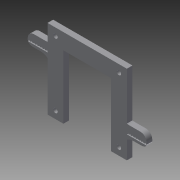
# Autodesk Inventor part: x carriage belt tensioner
Saved by Autodesk Inventor 2014 SP1 (Build 180222100, 222)
## iProperties
Created: 2014-10-23
Part Number: x carriage belt tensioner
Material: Generic
Document SubType Name: Modeling
Designer: Mon
Density: 1 g/cm^3
Appearance: Default
Author: Mon
Autodesk Inventor part; units mm, degrees
ref_plane "YZ Plane" through (0, 0, 0) normal (1, 0, 0) x (0, 1, 0)
ref_plane "XZ Plane" through (0, 0, 0) normal (0, 1, 0) x (-1, 0, 0)
ref_plane "XY Plane" through (0, 0, 0) normal (0, 0, 1) x (1, 0, 0)
sketch "Sketch1" plane through (0, 0, 0) normal (0, 1, 0) x (-1, 0, 0)
  line L0 (15.8278, -0.0229) -> (15.8278, 14.2578)
  arc A0 (15.8278, 14.2578) -> (10.4826, 16.0171) centre (10.4826, 7.0171) ccw
  line L1 (10.4826, 16.0171) -> (4.0229, 16.0171)
  arc A1 (0.0229, 18.0171) -> (4.0229, 16.0171) centre (4.0229, 21.0171) ccw
  line L2 (0.0229, 18.0171) -> (15.8278, 18.0171)
  line L3 (15.8278, 18.0171) -> (15.8278, 18.7671)
  line L4 (15.8278, 18.7671) -> (15.6604, 19.2271)
  line L5 (15.6604, 19.2271) -> (14.9004, 19.2271)
  line L6 (14.9004, 19.2271) -> (14.7329, 18.7671)
  line L7 (14.7329, 18.7671) -> (13.7978, 18.7671)
  line L8 (13.7978, 18.7671) -> (13.6304, 19.2271)
  line L9 (13.6304, 19.2271) -> (12.8704, 19.2271)
  line L10 (12.8704, 19.2271) -> (12.7029, 18.7671)
  line L11 (12.7029, 18.7671) -> (11.7678, 18.7671)
  line L12 (11.7678, 18.7671) -> (11.6004, 19.2271)
  line L13 (11.6004, 19.2271) -> (10.8404, 19.2271)
  line L14 (10.8404, 19.2271) -> (10.6729, 18.7671)
  line L15 (10.6729, 18.7671) -> (9.7378, 18.7671)
  line L16 (9.7378, 18.7671) -> (9.5704, 19.2271)
  line L17 (9.5704, 19.2271) -> (8.8104, 19.2271)
  line L18 (8.8104, 19.2271) -> (8.6429, 18.7671)
  line L19 (8.6429, 18.7671) -> (7.7078, 18.7671)
  line L20 (7.7078, 18.7671) -> (7.5404, 19.2271)
  line L21 (7.5404, 19.2271) -> (6.7804, 19.2271)
  line L22 (6.7804, 19.2271) -> (6.6129, 18.7671)
  line L23 (6.6129, 18.7671) -> (5.6778, 18.7671)
  line L24 (5.6778, 18.7671) -> (5.5104, 19.2271)
  line L25 (5.5104, 19.2271) -> (4.7504, 19.2271)
  line L26 (4.7504, 19.2271) -> (4.5829, 18.7671)
  line L27 (4.5829, 18.7671) -> (3.6478, 18.7671)
  line L28 (3.6478, 18.7671) -> (3.4804, 19.2271)
  line L29 (3.4804, 19.2271) -> (2.7204, 19.2271)
  line L30 (2.7204, 19.2271) -> (2.5529, 18.7671)
  line L31 (2.5529, 18.7671) -> (1.6178, 18.7671)
  line L32 (1.6178, 18.7671) -> (1.4504, 19.2271)
  line L33 (1.4504, 19.2271) -> (0.6904, 19.2271)
  line L34 (0.6904, 19.2271) -> (0.5229, 18.7671)
  line L35 (0.5229, 18.7671) -> (0.0229, 18.7671)
  line L36 (0.0229, 18.7671) -> (0.0229, 20.2271)
  arc A2 (5.0229, 25.2271) -> (0.0229, 20.2271) centre (5.0229, 20.2271) ccw
  line L37 (5.0229, 25.2271) -> (14.0269, 25.2271)
  line L38 (14.0269, 25.2271) -> (14.9274, 25.2583)
  line L39 (14.9274, 25.2583) -> (15.8278, 25.4494)
  line L40 (15.8278, 25.4494) -> (15.8278, 63.4771)
  line L41 (15.8278, 63.4771) -> (79.3278, 63.4771)
  line L42 (79.3278, 63.4771) -> (79.3278, 50.4494)
  line L43 (79.3278, 50.4494) -> (80.2012, 50.261)
  line L44 (80.2012, 50.261) -> (81.1287, 50.2271)
  line L45 (81.1287, 50.2271) -> (90.1326, 50.2271)
  arc A3 (95.1326, 45.2271) -> (90.1326, 50.2271) centre (90.1326, 45.2271) ccw
  line L46 (95.1326, 45.2271) -> (95.1326, 43.7671)
  line L47 (95.1326, 43.7671) -> (94.6326, 43.7671)
  line L48 (94.6326, 43.7671) -> (94.4652, 44.2271)
  line L49 (94.4652, 44.2271) -> (93.7052, 44.2271)
  line L50 (93.7052, 44.2271) -> (93.5378, 43.7671)
  line L51 (93.5378, 43.7671) -> (92.6026, 43.7671)
  line L52 (92.6026, 43.7671) -> (92.4352, 44.2271)
  line L53 (92.4352, 44.2271) -> (91.6752, 44.2271)
  line L54 (91.6752, 44.2271) -> (91.5078, 43.7671)
  line L55 (91.5078, 43.7671) -> (90.5726, 43.7671)
  line L56 (90.5726, 43.7671) -> (90.4052, 44.2271)
  line L57 (90.4052, 44.2271) -> (89.6452, 44.2271)
  line L58 (89.6452, 44.2271) -> (89.4778, 43.7671)
  line L59 (89.4778, 43.7671) -> (88.5426, 43.7671)
  line L60 (88.5426, 43.7671) -> (88.3752, 44.2271)
  line L61 (88.3752, 44.2271) -> (87.6152, 44.2271)
  line L62 (87.6152, 44.2271) -> (87.4478, 43.7671)
  line L63 (87.4478, 43.7671) -> (86.5126, 43.7671)
  line L64 (86.5126, 43.7671) -> (86.3452, 44.2271)
  line L65 (86.3452, 44.2271) -> (85.5852, 44.2271)
  line L66 (85.5852, 44.2271) -> (85.4178, 43.7671)
  line L67 (85.4178, 43.7671) -> (84.4826, 43.7671)
  line L68 (84.4826, 43.7671) -> (84.3152, 44.2271)
  line L69 (84.3152, 44.2271) -> (83.5552, 44.2271)
  line L70 (83.5552, 44.2271) -> (83.3878, 43.7671)
  line L71 (83.3878, 43.7671) -> (82.4526, 43.7671)
  line L72 (82.4526, 43.7671) -> (82.2852, 44.2271)
  line L73 (82.2852, 44.2271) -> (81.5252, 44.2271)
  line L74 (81.5252, 44.2271) -> (81.3578, 43.7671)
  line L75 (81.3578, 43.7671) -> (80.4226, 43.7671)
  line L76 (80.4226, 43.7671) -> (80.2552, 44.2271)
  line L77 (80.2552, 44.2271) -> (79.4952, 44.2271)
  line L78 (79.4952, 44.2271) -> (79.3278, 43.7671)
  line L79 (79.3278, 43.7671) -> (79.3278, 43.0171)
  line L80 (79.3278, 43.0171) -> (95.1326, 43.0171)
  arc A4 (91.1326, 41.0171) -> (95.1326, 43.0171) centre (91.1326, 46.0171) ccw
  line L81 (91.1326, 41.0171) -> (84.673, 41.0171)
  arc A5 (84.673, 41.0171) -> (79.3278, 39.2578) centre (84.673, 32.0171) ccw
  line L82 (79.3278, 39.2578) -> (79.3278, -0.0229)
  line L83 (79.3278, -0.0229) -> (66.6278, -0.0229)
  line L84 (66.6278, -0.0229) -> (66.6278, 50.7771)
  line L85 (66.6278, 50.7771) -> (28.5278, 50.7771)
  line L86 (28.5278, 50.7771) -> (28.5278, -0.0229)
  line L87 (28.5278, -0.0229) -> (15.8278, -0.0229)
  circle A6 centre (22.1778, 5.9146) radius 1.75
  circle A7 centre (22.1778, 57.5396) radius 1.75
  circle A8 centre (72.9778, 57.5396) radius 1.75
  circle A9 centre (72.9778, 5.9146) radius 1.75
  point P0 (0, 0)
  constraints: 176 end point, 12 point on circle, 10 centre point
extrude "Extrusion1" add sketch "Sketch1" along normal blind 4.5
body "Solid1"
